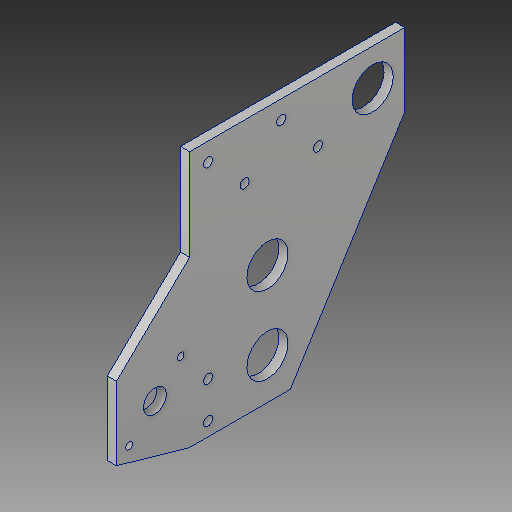
# Autodesk Inventor part: 15102898-16-P-0302
Saved by Autodesk Inventor 2017 (Build 210142000, 142)
## iProperties
Created: 2016-10-02
Part Number: 15102898-16-P-0302
Material: Aluminum 6061
Document SubType Name: Sheet Metal
Designer: gus
Density: 2.7 g/cm^3
Appearance: Aluminum - Flat
Sheet Metal Rule: Default
Mass: 400.129 g
Surface Area: 538.272 cm^2
Volume: 148.196 cm^3
Author: gus
Autodesk Inventor part; units mm, degrees
ref_plane "YZ Plane" through (0, 0, 0) normal (1, 0, 0) x (0, 1, 0)
ref_plane "XZ Plane" through (0, 0, 0) normal (0, 1, 0) x (-1, 0, 0)
ref_plane "XY Plane" through (0, 0, 0) normal (0, 0, 1) x (1, 0, 0)
sketch "Sketch1" plane through (0, 0, 0) normal (1, 0, 0) x (0, 1, 0)
  line L0 (0, 0) -> (63.5, 0)
  line L1 (63.5, 0) -> (63.5, -149.225)
  line L2 (63.5, -149.225) -> (12.7, -149.225)
  circle A0 centre (-31.75, -53.975) radius 14.2875
  line L3 (63.5, -25.4) -> (-43.502, -25.4) construction
  circle A1 centre (50.8, -12.7) radius 3.175
  circle A2 centre (-104.775, -12.7) radius 3.175
  line L4 (12.7, -149.225) -> (-114.3, -69.85)
  line L5 (-114.3, -69.85) -> (-114.3, 0)
  line L6 (-114.3, 0) -> (0, 0) construction
  circle A3 centre (-85.725, -53.975) radius 14.2875
  line L7 (-53.2384, 0) -> (-95.25, 0)
  line L8 (-95.25, 0) -> (-95.25, 45.1866) construction
  line L9 (-95.25, 45.1866) -> (-53.2384, 45.1866) construction
  line L10 (-53.2384, 45.1866) -> (-53.2384, 0) construction
  line L11 (-95.25, 45.1866) -> (-114.3, 0) construction
  line L12 (-53.2384, 45.1866) -> (0, 0) construction
  circle A4 centre (-56.3011, 6.2145) radius 2.3813
  circle A5 centre (-92.2105, 42.1471) radius 2.3813
  line L13 (0, 0) -> (-49.0855, 50.8)
  line L14 (-49.0855, 50.8) -> (-99.8855, 50.8)
  line L15 (-99.8855, 50.8) -> (-114.3, 0)
  circle A6 centre (-74.2558, 24.1808) radius 7.9375
  line L16 (-92.2105, 42.1471) -> (-74.2558, 24.1808) construction
  line L17 (-74.2558, 24.1808) -> (-56.3011, 6.2145) construction
  circle A7 centre (38.1, -127) radius 14.2875
  circle A8 centre (22.225, -88.9) radius 3.175
  circle A9 centre (50.8, -63.5) radius 3.175
  circle A10 centre (25.4, -38.1) radius 3.175
  circle A11 centre (-79.375, -12.7) radius 3.175
  dimension "d1" = 28.575
  dimension "d2" = 63.5
  dimension "d6" = 25.4
  dimension "d7" = 6.35
  dimension "d8" = 6.35
  dimension "d9" = 12.7
  dimension "d10" = 12.7
  dimension "d12" = 12.7
  dimension "d17" = 50.8
  dimension "d18" = 114.3
  dimension "d19" = 9.525
  dimension "d20" = 53.975
  dimension "d21" = 28.575
  dimension "d24" = 53.975
  dimension "d25" = 69.85
  dimension "d26" = 53.975
  dimension "d27" = 149.225
  dimension "d28" = 107.002
  dimension "d29" = 42.0116
  dimension "d30" = 19.05
  dimension "d31" = 45.1866
  dimension "d32" = 50.8
  dimension "d33" = 4.7625
  dimension "d34" = 3.0395
  dimension "d35" = 3.0395
  dimension "d36" = 6.2145
  dimension "d37" = 50.8
  dimension "d38" = 50.8
  dimension "d39" = 4.1529
  dimension "d40" = 15.875
  dimension "d42" = 22.225
  dimension "d43" = 25.4
  dimension "d44" = 28.575
  dimension "d45" = 6.35
  dimension "d46" = 6.35
  dimension "d47" = 6.35
  dimension "d48" = 38.1
  dimension "d49" = 38.1
  dimension "d50" = 41.275
  dimension "d51" = 12.7
  dimension "d52" = 63.5
  dimension "d53" = 88.9
  dimension "d54" = 6.35
  dimension "d55" = 12.7
  dimension "d56" = 25.4
  constraints: 36 end point, 12 centre point, 3 collinear, 3 horizontal, 3 parallel, 3 perpendicular, 2 equal radius, 2 point on line
  measures "d1" diameter of A0
  measures "d2" distance of L0.start L0.end
  measures "d6" distance between parallel lines of L0 L3
  measures "d7" diameter of A1
  measures "d8" diameter of A2
  measures "d9" distance from line of L3 A2.centre
  measures "d10" distance from line of L3 A1.centre
  measures "d12" distance from line of L1 A1.centre
  measures "d17" distance of L1.end L2.end
  measures "d18" distance from line of L0.start L5
  measures "d19" distance from line of L5 A2.centre
  measures "d20" distance from line of L6 A3.centre
  measures "d21" distance from line of L5 A3.centre
  measures "d24" distance from line of L0 A0.centre
  measures "d25" distance of L4.end L5.end
  measures "d26" distance of A3.centre A0.centre
  measures "d27" distance of L0.end L1.end
  measures "d28" distance of L3.start L3.end
  measures "d29" distance between parallel lines of L10 L8
  measures "d30" distance between parallel lines of L5 L8
  measures "d31" distance between parallel lines of L7 L9
  measures "d32" distance of L16.start L17.end
  measures "d33" diameter of A4
  measures "d34" distance from line of L9 L16.start
  measures "d35" distance from line of L8 L16.start
  measures "d36" distance from line of L7 L17.end
  measures "d37" distance of L13.end L14.end
  measures "d38" distance between parallel lines of L6 L14
  measures "d39" distance from line of L10 L13.end
  measures "d40" diameter of A6
  measures "d42" distance from line of L2 A7.centre
  measures "d43" distance from line of L1 A7.centre
  measures "d44" diameter of A7
  measures "d45" diameter of A8
  measures "d46" diameter of A9
  measures "d47" diameter of A10
  measures "d48" distance from line of L1 A10.centre
  measures "d49" distance from line of L0 A10.centre
  measures "d50" distance from line of L1 A8.centre
  measures "d51" distance from line of L1 A9.centre
  measures "d52" distance from line of L0 A9.centre
  measures "d53" distance from line of L0 A8.centre
  measures "d54" diameter of A11
  measures "d55" distance from line of L6 A11.centre
  measures "d56" distance of A2.centre A11.centre
extrude "Extrusion1" add sketch "Sketch1" along normal blind 6.35 contours L0 L1 L2 L4 L5 L15 L14 L13 | A3 | A4 | A5 | A6 | A7 | A8 | A9 | A10 | A11
extrude "Extrusion2" cut sketch "Sketch1" along normal blind 25.4 contours A3 | A4 | A5 | A6 | A7 | A8 | A9 | A10 | A11
equation "\"BendRadius\" = Thickness"
equation "\"BendReliefWidth\" = Thickness"
equation "\"BendReliefDepth\" = 0.5 * Thickness"
equation "\"CornerReliefSize\" = 4 * Thickness"
equation "\"MinimumRemnant\" = 2 * Thickness"
equation "\"TransitionRadius\" = BendRadius"
equation "\"JacobiRadiusSize\" = Thickness"
equation "\"GapSize\" = Thickness"
equation "\"Thickness\" = 3.048"
body "Solid1"
